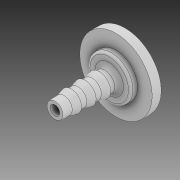
# Autodesk Inventor part: Bottle Adapter
Saved by Autodesk Inventor 2020 (Build 240168000, 168)
## iProperties
Created: 2020-08-02
Part Number: Bottle Adapter
Material: Generic
Document SubType Name: Modeling
Designer: DDeGo
Density: 1 g/cm^3
Appearance: Default
Author: DDeGo
Autodesk Inventor part; units mm, degrees
ref_plane "YZ Plane" through (0, 0, 0) normal (1, 0, 0) x (0, 1, 0)
ref_plane "XZ Plane" through (0, 0, 0) normal (0, 1, 0) x (-1, 0, 0)
ref_plane "XY Plane" through (0, 0, 0) normal (0, 0, 1) x (1, 0, 0)
sketch "Sketch1" plane through (0, 0, 0) normal (1, 0, 0) x (0, 1, 0)
  line L0 (0, 0) -> (1.05, 0) construction
  line L1 (2.2, 3.5) -> (2.118, 5.6871)
  line L2 (1.75, 15.5) -> (1.05, 15.5)
  line L3 (1.05, 15.5) -> (1.05, 0)
  line L4 (0, 0) -> (0, 15.5) construction
  line L5 (0, 15.5) -> (1.05, 15.5) construction
  line L6 (1.05, 0) -> (4.4824, 0)
  line L7 (1.825, 13.5) -> (2.2852, 11.9107)
  line L8 (2.2852, 11.9107) -> (1.8852, 11.8957)
  line L9 (1.9414, 10.3957) -> (2.4016, 8.8064)
  line L10 (2.4016, 8.8064) -> (2.0016, 8.7914)
  line L11 (2.0578, 7.2914) -> (2.518, 5.7021)
  line L12 (2.518, 5.7021) -> (2.118, 5.6871)
  line L13 (2.2, 3.5) -> (4.7625, 3.5)
  line L14 (4.7625, 3.5) -> (4.7625, 2)
  line L15 (4.7625, 2) -> (8, 2)
  line L16 (8, 2) -> (8, 0)
  line L17 (8, 0) -> (4.4824, 0)
  line L18 (1.8852, 11.8957) -> (1.825, 13.5) construction
  line L19 (1.825, 13.5) -> (1.75, 15.5)
  line L20 (1.9414, 10.3957) -> (1.8852, 11.8957)
  line L21 (2.0016, 8.7914) -> (1.9414, 10.3957) construction
  line L22 (2.0578, 7.2914) -> (2.0016, 8.7914)
  line L23 (2.118, 5.6871) -> (2.0578, 7.2914) construction
  dimension "d0" = 1.75
  dimension "d1" = 0.7
  dimension "d2" = 2.2
  dimension "d3" = 0.4
  dimension "d5" = 12
  dimension "d6" = 2
  dimension "d7" = 1.5
  dimension "d9" = 1.5
  dimension "d10" = 4.7625
  dimension "d11" = 1.5
  dimension "d12" = 2
  dimension "d13" = 8
  dimension "d14" = 14
  constraints: 48 end point, 27 perpendicular, 4 horizontal, 4 parallel, 2 vertical, 1 point on line
  measures "d0" distance of L4.end L2.start
  measures "d1" distance of L2.start L2.end
  measures "d2" distance from line of L4 L1.start
  measures "d3" horizontal distance of L7.end L8.end
  measures "d5" vertical distance of L1.start L2.start
  measures "d6" vertical distance of L2.end L7.start
  measures "d7" vertical distance of L8.end L9.start
  measures "d9" vertical distance of L10.end L11.start
  measures "d10" distance between parallel lines of L4 L14
  measures "d11" distance of L13.end L14.end
  measures "d12" distance of L15.end L16.end
  measures "d13" distance between parallel lines of L4 L16
  measures "d14" angle of L7 L18
revolve "Revolution1" add sketch "Sketch1" angle 360 about axis through (0, 0, 0) along (0, 0, 1)
fillet "Fillet1" radius 2 1 edges at (0, -1.05, 0)
fillet "Fillet2" radius 0.5 1 edges at (0, -4.7625, 3.5)
fillet "Fillet3" radius 1 1 edges at (0, -2.2, 3.5)
body "Solid1"
